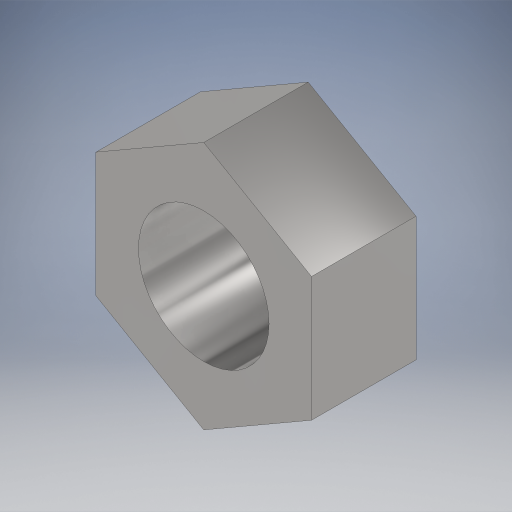
# Autodesk Inventor part: Гайка М6
Saved by Autodesk Inventor 2023 (Build 270158000, 158)
## iProperties
Created: 2023-01-04
Part Number: Гайка М6
Material: Типовые
Document SubType Name: Modeling
Designer: Admin
Density: 1 g/cm^3
Appearance: По умолчанию
Author: Admin
Autodesk Inventor part; units mm, degrees
ref_plane "YZ Plane" through (0, 0, 0) normal (1, 0, 0) x (0, 1, 0)
ref_plane "XZ Plane" through (0, 0, 0) normal (0, 1, 0) x (-1, 0, 0)
ref_plane "XY Plane" through (0, 0, 0) normal (0, 0, 1) x (1, 0, 0)
sketch "Эскиз1" plane through (0, 0, 0) normal (0, 0, 1) x (1, 0, 0)
  line L0 (0, 5.7158) -> (4.95, 2.8579)
  line L1 (4.95, 2.8579) -> (4.95, -2.8579)
  line L2 (4.95, -2.8579) -> (0, -5.7158)
  line L3 (0, -5.7158) -> (-4.95, -2.8579)
  line L4 (-4.95, -2.8579) -> (-4.95, 2.8579)
  line L5 (-4.95, 2.8579) -> (0, 5.7158)
  circle A0 centre (0, 0) radius 3
  dimension "d0" = 6
  dimension "d1" = 9.9
  constraints: 12 end point, 2 coincident, 1 centre point, 1 vertical, 13 other
  measures "d0" diameter of A0
  measures "d1" distance between parallel lines of L4 L1
extrude "Выдавливание1" add sketch "Эскиз1" along normal blind 4.8
